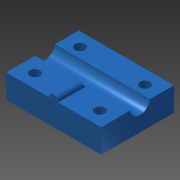
# Autodesk Inventor part: YMotorCapLeft
Saved by Autodesk Inventor 2015 (Build 190159000, 159)
## iProperties
Created: 2014-08-15
Part Number: YMotorCapLeft
Material: ABS Plastic
Document SubType Name: Modeling
Designer: t_clevj
Density: 1.06 g/cm^3
Appearance: Cyan
Author: t_clevj
Autodesk Inventor part; units mm, degrees
ref_plane "YZ Plane" through (0, 0, 0) normal (1, 0, 0) x (0, 1, 0)
ref_plane "XZ Plane" through (0, 0, 0) normal (0, 1, 0) x (-1, 0, 0)
ref_plane "XY Plane" through (0, 0, 0) normal (0, 0, 1) x (1, 0, 0)
sketch "Sketch1" plane through (0, 0, 0) normal (0, 0, 1) x (1, 0, 0)
  line L0 (0, 0) -> (38, 0)
  line L1 (38, 0) -> (38, 29)
  line L2 (38, 29) -> (0, 29)
  line L3 (0, 29) -> (0, 0)
  dimension "d0" = 38
  dimension "d1" = 29
  constraints: 8 end point, 2 parallel, 1 horizontal, 1 perpendicular
  measures "d0" distance of L2.end L1.end
  measures "d1" distance of L1.end L0.end
extrude "Extrusion1" add sketch "Sketch1" along normal blind 9.5
sketch "Sketch2" plane through (0, 0, 0) normal (-1, 0, 0) x (0, 0, 1)
  line L0 (9.5, 29) -> (9.5, 0) projected
  line L1 (0, 29) -> (9.5, 29) projected
  circle A0 centre (10, 15.5) radius 4
  dimension "d4" = 8
  dimension "d5" = 0.5
  dimension "d6" = 13.5
  constraints: 1 centre point
  measures "d4" diameter of A0
  measures "d5" distance from line of L0 A0.centre
  measures "d6" distance from line of L1 A0.centre
extrude "Extrusion2" cut sketch "Sketch2" against normal up to surface (38 mm away)
sketch "Sketch3" plane through (0, 0, 0) normal (0, 0, -1) x (-1, 0, 0)
  line L0 (0, 0) -> (-38, 0) projected
  line L1 (0, 29) -> (0, 0) projected
  point P0 (-6, 23.5)
  point P1 (-32, 23.5)
  point P2 (-32, 5.5)
  point P3 (-6, 5.5)
  dimension "d9" = 6
  dimension "d10" = 32
  dimension "d11" = 5.5
  dimension "d12" = 23.5
  constraints: 2 horizontal alignment, 2 vertical alignment
  measures "d9" distance from line of L1 point (-6, 23.5)
  measures "d10" distance from line of point (-32, 23.5) L1
  measures "d11" distance from line of L0 point (-6, 5.5)
  measures "d12" distance from line of L0 point (-6, 23.5)
hole "Hole1" at (6, 23.5, 0) at (32, 23.5, 0) at (32, 5.5, 0) at (6, 5.5, 0) direction (0, 0, 1) diameter 4 depth 9.5 tip angle 118 counterbore diameter 7 counterbore depth 3.2
sketch "Sketch4" plane through (0, 0, 0) normal (0, -1, 0) x (1, 0, 0)
  line L0 (0, 9.5) -> (38, 9.5) projected
  line L1 (0, 0) -> (0, 9.5) projected
  circle A0 centre (19, 9.5) radius 1.8
  dimension "d20" = 3.6
  dimension "d22" = 19
  dimension "d23" = 0
  constraints: 1 centre point
  measures "d20" diameter of A0
  measures "d22" distance from line of L1 A0.centre
  measures "d23" distance from line of L0 A0.centre
extrude "Extrusion3" add sketch "Sketch4" against normal blind 10
fillet "Fillet2" radius 1.5 1 edges at (19, 10, 9.5)
body "Solid1"
